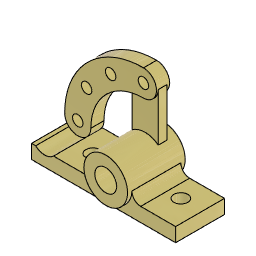
Exercise-11 v0 (Autodesk Fusion 360 design; units mm, degrees)
Autodesk Fusion 360 part; units mm, degrees
sketch "Sketch2" plane through (0, 0, 0) normal (0, 1, 0) x (1, 0, 0)
  line L0 (82.5, -8) -> (-82.5, -8)
  line L1 (-82.5, -8) -> (-82.5, 8)
  line L2 (-82.5, 8) -> (82.5, 8)
  line L3 (82.5, 8) -> (82.5, -8)
  line L4 (82.5, -8) -> (-82.5, 8) construction
  line L5 (-82.5, -8) -> (82.5, 8) construction
  circle A0 centre (7.5, -19) radius 12.5
  circle A1 centre (7.5, -19) radius 25
  arc A2 (-82.5, -19) -> (7.7051, -108.9998) centre (7.5, -19) ccw
  arc A3 (-52.5, -19) -> (7.6367, -78.9998) centre (7.5, -19) ccw
  circle A4 centre (7.6709, -93.9998) radius 15
  circle A5 centre (-67.5, -19) radius 15
  line L6 (22.6709, -93.9998) -> (22.6709, -38.8707)
  line L7 (-7.3291, -93.9998) -> (-7.3291, -39.127)
  circle A6 centre (7.6709, -93.9998) radius 6
  circle A7 centre (-29.8519, -84.0372) radius 6
  circle A8 centre (-57.3663, -56.6479) radius 6
  circle A9 centre (-67.4998, -19.1709) radius 6
  dimension "d12" = 165
  dimension "d13" = 16
  dimension "d14" = 25
  dimension "d15" = 50
  dimension "d16" = 7.5
  dimension "d17" = 27
  dimension "d18" = 60
  dimension "d19" = 90
  dimension "d20" = 30
  dimension "d21" = 12
  dimension "d23" = -90
  constraint horizontal L0
  constraint perpendicular L0 L1
  constraint parallel L0 L2
  constraint parallel L1 L3
  constraint coincident L4 origin
  constraint coincident L5 origin
  constraint concentric A0 A1
  constraint coincident A0.centre A1.centre
  constraint coincident A2.end A4
  constraint tangent A2 A4
  constraint coincident A3.end A4
  constraint coincident A2.start A5
  constraint tangent A2 A5
  constraint coincident A3.start A5
  constraint coincident A4 L6.start
  constraint coincident A1 L6.end
  constraint vertical L6
  constraint coincident A4 L7.start
  constraint coincident A1 L7.end
  constraint parallel L6 L7
  constraint tangent A4 L6
  constraint tangent A4 L7
  constraint concentric A4 A6
  measures "d12" distance of L1.end L2.end
  measures "d13" distance of L0.end L1.end
  measures "d14" diameter of A0
  measures "d15" diameter of A1
  measures "d16" horizontal distance of origin A0.centre
  measures "d17" distance of L2 A0.centre
  measures "d18" radius of A3
  measures "d19" radius of A2
  measures "d20" distance of L6 L7
  measures "d21" diameter of A6
extrude "Extrude1" add sketch "Sketch2" along normal mid plane 56 contours L0 L1 L2 L3 A1 A5
extrude "Extrude2" add sketch "Sketch2" along normal mid plane 66 contours L0 A0 A1 | L0 A0 A1
extrude "Extrude3" add sketch "Sketch2" along normal blind 15 from surface at 10 contours L0 A5 | L0 A5 | A4 | A2 A3 A4 A5 L7 | A3 A4 L7
extrude "Extrude4" add sketch "Sketch2" along normal blind 10 from surface at 12 contours A1 A3 A4 L6 L7
hole "Hole1" at (57.5, 3, 8) direction (0, 0, -1) diameter 16 end through all
hole "Hole2" at (-37.302, -3, 8) direction (0, 0, -1) diameter 16 end through all
fillet "Fillet1" radius 10 1 edges at (29.9499, 0, 8)
